Autodesk Inventor part; units mm, degrees
(part 3 of 3)
sketch "Эскиз6" plane through (0, 2, 0) normal (0, 1, 0) x (1, 0, 0)
  circle A0 centre (0, -40) radius 1.6 construction
  circle A1 centre (-46, 0) radius 1.6 construction
  circle A2 centre (46, 0) radius 1.6 construction
  line L0 (-6.2595, 46.1335) -> (-19.2746, 46.1335) construction
  arc A3 (-19.2746, 46.1335) -> (-21.6698, 47.1257) centre (-21.9203, 43.1335) ccw construction
  line L1 (-21.6698, 47.1257) -> (-42.4264, 67.8823) construction
  line L2 (-42.4264, 67.8823) -> (-34.2947, 76.014) construction
  arc A4 (-34.2947, 76.014) -> (-34.2947, 83.085) centre (-37.8302, 79.5495) ccw construction
  line L3 (-34.2947, 83.085) -> (-38.3892, 87.1795) construction
  arc A5 (-37.7453, 90.4395) -> (-38.3892, 87.1795) centre (-36.975, 88.5938) ccw construction
  arc A6 (-25.8102, 94.5401) -> (-37.7453, 90.4395) centre (0, 0) ccw construction
  arc A7 (-25.8102, 94.5401) -> (-20.7476, 95.7786) centre (-24, 98.1071) ccw construction
  arc A8 (20.7476, 95.7786) -> (-20.7476, 95.7786) centre (0, 0) ccw construction
  arc A9 (20.7476, 95.7786) -> (25.8102, 94.5401) centre (24, 98.1071) ccw construction
  arc A10 (37.7453, 90.4395) -> (25.8102, 94.5401) centre (0, 0) ccw construction
  arc A11 (38.3892, 87.1795) -> (37.7453, 90.4395) centre (36.975, 88.5938) ccw construction
  line L4 (38.3892, 87.1795) -> (34.2947, 83.085) construction
  arc A12 (34.2947, 83.085) -> (34.2947, 76.014) centre (37.8302, 79.5495) ccw construction
  line L5 (34.2947, 76.014) -> (42.4264, 67.8823) construction
  line L6 (42.4264, 67.8823) -> (21.6698, 47.1257) construction
  arc A13 (21.6698, 47.1257) -> (19.2746, 46.1335) centre (21.9203, 43.1335) ccw construction
  line L7 (19.2746, 46.1335) -> (6.2595, 46.1335) construction
  arc A14 (3.5768, 47.7906) -> (6.2595, 46.1335) centre (6.2595, 49.1335) ccw construction
  arc A15 (3.5768, 47.7906) -> (-3.5768, 47.7906) centre (0, 46) ccw construction
  arc A16 (-6.2595, 46.1335) -> (-3.5768, 47.7906) centre (-6.2595, 49.1335) ccw construction
  arc A17 (48.6481, 93.0503) -> (-48.6481, 93.0503) centre (0, 0) ccw construction
  arc A18 (-48.6481, 93.0503) -> (-49.3795, 88.2704) centre (-47.2582, 90.3917) ccw construction
  line L8 (-49.3795, 88.2704) -> (-46.3155, 85.2064) construction
  arc A19 (-46.3155, 73.8927) -> (-46.3155, 85.2064) centre (-51.9723, 79.5495) ccw construction
  line L9 (-46.3155, 73.8927) -> (-73.8927, 46.3155) construction
  arc A20 (-85.2064, 46.3155) -> (-73.8927, 46.3155) centre (-79.5495, 51.9723) ccw construction
  line L10 (-85.2064, 46.3155) -> (-88.2704, 49.3795) construction
  arc A21 (-88.2704, 49.3795) -> (-93.0503, 48.6481) centre (-90.3917, 47.2582) ccw projected
  arc A22 (-93.0503, 48.6481) -> (-93.0503, -48.6481) centre (0, 0) ccw construction
  arc A23 (-93.0503, -48.6481) -> (-88.2704, -49.3795) centre (-90.3917, -47.2582) ccw projected
  line L11 (-88.2704, -49.3795) -> (-85.2064, -46.3155) construction
  arc A24 (-73.8927, -46.3155) -> (-85.2064, -46.3155) centre (-79.5495, -51.9723) ccw construction
  line L12 (-73.8927, -46.3155) -> (-46.3155, -73.8927) construction
  arc A25 (-46.3155, -85.2064) -> (-46.3155, -73.8927) centre (-51.9723, -79.5495) ccw construction
  line L13 (-46.3155, -85.2064) -> (-49.3795, -88.2704) construction
  arc A26 (-49.3795, -88.2704) -> (-48.6481, -93.0503) centre (-47.2582, -90.3917) ccw construction
  arc A27 (-48.6481, -93.0503) -> (-45.42, -94.668) centre (0, 0) ccw construction
  arc A28 (-45.42, -94.668) -> (-43.0355, -94.1655) centre (-44.5548, -92.8648) ccw construction
  line L14 (-43.0355, -94.1655) -> (-18.3802, -65.3664) construction
  arc A29 (-17.477, -64.7643) -> (-18.3802, -65.3664) centre (-16.8609, -66.6671) ccw construction
  line L15 (-17.477, -64.7643) -> (-0.6161, -59.3045) construction
  arc A30 (0.6161, -59.3045) -> (-0.6161, -59.3045) centre (0, -61.2072) ccw construction
  line L16 (0.6161, -59.3045) -> (17.477, -64.7643) construction
  arc A31 (18.3802, -65.3664) -> (17.477, -64.7643) centre (16.8609, -66.6671) ccw construction
  line L17 (18.3802, -65.3664) -> (43.0355, -94.1655) construction
  arc A32 (43.0355, -94.1655) -> (45.42, -94.668) centre (44.5548, -92.8648) ccw construction
  arc A33 (45.42, -94.668) -> (48.6481, -93.0503) centre (0, 0) ccw construction
  arc A34 (48.6481, -93.0503) -> (49.3795, -88.2704) centre (47.2582, -90.3917) ccw construction
  line L18 (49.3795, -88.2704) -> (46.3155, -85.2064) construction
  arc A35 (46.3155, -73.8927) -> (46.3155, -85.2064) centre (51.9723, -79.5495) ccw construction
  line L19 (46.3155, -73.8927) -> (73.8927, -46.3155) construction
  arc A36 (85.2064, -46.3155) -> (73.8927, -46.3155) centre (79.5495, -51.9723) ccw construction
  line L20 (85.2064, -46.3155) -> (88.2704, -49.3795) construction
  arc A37 (88.2704, -49.3795) -> (93.0503, -48.6481) centre (90.3917, -47.2582) ccw construction
  arc A38 (93.0503, -48.6481) -> (93.0503, 48.6481) centre (0, 0) ccw construction
  arc A39 (93.0503, 48.6481) -> (88.2704, 49.3795) centre (90.3917, 47.2582) ccw construction
  line L21 (88.2704, 49.3795) -> (85.2064, 46.3155) construction
  arc A40 (73.8927, 46.3155) -> (85.2064, 46.3155) centre (79.5495, 51.9723) ccw construction
  line L22 (73.8927, 46.3155) -> (46.3155, 73.8927) construction
  arc A41 (46.3155, 85.2064) -> (46.3155, 73.8927) centre (51.9723, 79.5495) ccw construction
  line L23 (46.3155, 85.2064) -> (49.3795, 88.2704) construction
  arc A42 (49.3795, 88.2704) -> (48.6481, 93.0503) centre (47.2582, 90.3917) ccw construction
  circle A43 centre (-24, 98.1071) radius 1.6 construction
  arc A44 (47.7906, -3.5768) -> (46.1335, -6.2595) centre (49.1335, -6.2595) ccw construction
  arc A45 (47.7906, -3.5768) -> (47.7906, 3.5768) centre (46, 0) ccw construction
  arc A46 (46.1335, 6.2595) -> (47.7906, 3.5768) centre (49.1335, 6.2595) ccw construction
  line L24 (46.1335, 6.2595) -> (46.1335, 19.2746) construction
  arc A47 (46.1335, 19.2746) -> (47.1257, 21.6698) centre (43.1335, 21.9203) ccw construction
  line L25 (47.1257, 21.6698) -> (67.8823, 42.4264) construction
  line L26 (67.8823, 42.4264) -> (76.014, 34.2947) construction
  arc A48 (76.014, 34.2947) -> (83.085, 34.2947) centre (79.5495, 37.8302) ccw construction
  line L27 (83.085, 34.2947) -> (87.1795, 38.3892) construction
  arc A49 (90.4395, 37.7453) -> (87.1795, 38.3892) centre (88.5938, 36.975) ccw construction
  arc A50 (97.9653, 2.6059) -> (90.4395, 37.7453) centre (0, 0) ccw construction
  arc A51 (97.9653, 2.6059) -> (97.9653, -2.6059) centre (101, 0) ccw construction
  arc A52 (90.4395, -37.7453) -> (97.9653, -2.6059) centre (0, 0) ccw construction
  arc A53 (87.1795, -38.3892) -> (90.4395, -37.7453) centre (88.5938, -36.975) ccw construction
  line L28 (87.1795, -38.3892) -> (83.085, -34.2947) construction
  arc A54 (83.085, -34.2947) -> (76.014, -34.2947) centre (79.5495, -37.8302) ccw construction
  line L29 (76.014, -34.2947) -> (67.8823, -42.4264) construction
  line L30 (67.8823, -42.4264) -> (47.1257, -21.6698) construction
  arc A55 (47.1257, -21.6698) -> (46.1335, -19.2746) centre (43.1335, -21.9203) ccw construction
  line L31 (46.1335, -19.2746) -> (46.1335, -6.2595) construction
  circle A56 centre (101, 0) radius 1.6 construction
  circle A57 centre (-101, 0) radius 1.6 construction
  arc A58 (-47.7906, 3.5768) -> (-46.1335, 6.2595) centre (-49.1335, 6.2595) ccw construction
  arc A59 (-47.7906, 3.5768) -> (-47.7906, -3.5768) centre (-46, 0) ccw construction
  arc A60 (-46.1335, -6.2595) -> (-47.7906, -3.5768) centre (-49.1335, -6.2595) ccw construction
  line L32 (-46.1335, -6.2595) -> (-46.1335, -19.2746) construction
  arc A61 (-46.1335, -19.2746) -> (-47.1257, -21.6698) centre (-43.1335, -21.9203) ccw construction
  line L33 (-47.1257, -21.6698) -> (-67.8823, -42.4264) construction
  line L34 (-67.8823, -42.4264) -> (-76.014, -34.2947) construction
  arc A62 (-76.014, -34.2947) -> (-83.085, -34.2947) centre (-79.5495, -37.8302) ccw construction
  line L35 (-83.085, -34.2947) -> (-87.1795, -38.3892) construction
  arc A63 (-90.4395, -37.7453) -> (-87.1795, -38.3892) centre (-88.5938, -36.975) ccw construction
  arc A64 (-97.9653, -2.6059) -> (-90.4395, -37.7453) centre (0, 0) ccw construction
  arc A65 (-97.9653, -2.6059) -> (-97.9653, 2.6059) centre (-101, 0) ccw construction
  arc A66 (-90.4395, 37.7453) -> (-97.9653, 2.6059) centre (0, 0) ccw construction
  arc A67 (-87.1795, 38.3892) -> (-90.4395, 37.7453) centre (-88.5938, 36.975) ccw construction
  line L36 (-87.1795, 38.3892) -> (-83.085, 34.2947) construction
  arc A68 (-83.085, 34.2947) -> (-76.014, 34.2947) centre (-79.5495, 37.8302) ccw construction
  line L37 (-76.014, 34.2947) -> (-67.8823, 42.4264) construction
  line L38 (-67.8823, 42.4264) -> (-47.1257, 21.6698) construction
  arc A69 (-47.1257, 21.6698) -> (-46.1335, 19.2746) centre (-43.1335, 21.9203) ccw construction
  line L39 (-46.1335, 19.2746) -> (-46.1335, 6.2595) construction
  circle A70 centre (45.1111, -90.3659) radius 1.6 construction
  circle A71 centre (45.1111, 90.3659) radius 1.6 construction
  circle A72 centre (90.3659, 45.1111) radius 1.6 construction
  circle A73 centre (-45.1111, -90.3659) radius 1.6 construction
  circle A74 centre (90.3659, -45.1111) radius 1.6 construction
  circle A75 centre (-45.1111, 90.3659) radius 1.6 construction
  circle A76 centre (-90.3659, 45.1111) radius 1.6 construction
  circle A77 centre (-90.3659, -45.1111) radius 1.6 construction
  line L40 (63.6396, 46.669) -> (43.8406, 26.8701) construction
  arc A78 (41.0122, 26.8701) -> (43.8406, 26.8701) centre (42.4264, 28.2843) ccw construction
  line L41 (41.0122, 26.8701) -> (26.8701, 41.0122) construction
  arc A79 (26.8701, 43.8406) -> (26.8701, 41.0122) centre (28.2843, 42.4264) ccw construction
  line L42 (26.8701, 43.8406) -> (46.669, 63.6396) construction
  line L43 (46.669, 63.6396) -> (63.6396, 46.669) construction
  line L44 (-46.669, 63.6396) -> (-26.8701, 43.8406) construction
  arc A80 (-26.8701, 41.0122) -> (-26.8701, 43.8406) centre (-28.2843, 42.4264) ccw construction
  line L45 (-26.8701, 41.0122) -> (-41.0122, 26.8701) construction
  arc A81 (-43.8406, 26.8701) -> (-41.0122, 26.8701) centre (-42.4264, 28.2843) ccw construction
  line L46 (-43.8406, 26.8701) -> (-63.6396, 46.669) construction
  line L47 (-63.6396, 46.669) -> (-46.669, 63.6396) construction
  line L48 (-63.6396, -46.669) -> (-43.8406, -26.8701) construction
  arc A82 (-41.0122, -26.8701) -> (-43.8406, -26.8701) centre (-42.4264, -28.2843) ccw construction
  line L49 (-41.0122, -26.8701) -> (-26.8701, -41.0122) construction
  arc A83 (-26.8701, -43.8406) -> (-26.8701, -41.0122) centre (-28.2843, -42.4264) ccw construction
  line L50 (-26.8701, -43.8406) -> (-46.669, -63.6396) construction
  line L51 (-46.669, -63.6396) -> (-63.6396, -46.669) construction
  line L52 (-42.4264, -67.8823) -> (-21.6698, -47.1257) construction
  arc A84 (-21.6698, -47.1257) -> (-19.2746, -46.1335) centre (-21.9203, -43.1335) ccw construction
  line L53 (-19.2746, -46.1335) -> (19.2746, -46.1335) construction
  arc A85 (19.2746, -46.1335) -> (21.6698, -47.1257) centre (21.9203, -43.1335) ccw construction
  line L54 (21.6698, -47.1257) -> (42.4264, -67.8823) construction
  line L55 (42.4264, -67.8823) -> (37.1244, -73.1843) construction
  arc A86 (34.1909, -73.0707) -> (37.1244, -73.1843) centre (35.7102, -71.7701) ccw construction
  line L56 (34.1909, -73.0707) -> (25.4187, -62.8242) construction
  arc A87 (24.842, -61.8893) -> (25.4187, -62.8242) centre (28.1154, -60.5155) ccw construction
  line L57 (24.842, -61.8893) -> (23.8313, -59.4808) construction
  arc A88 (23.8313, -59.4808) -> (21.0049, -57.3328) centre (20.5578, -60.8546) ccw construction
  line L58 (21.0049, -57.3328) -> (15.1585, -56.5907) construction
  arc A89 (14.5119, -56.4463) -> (15.1585, -56.5907) centre (15.6055, -53.069) ccw construction
  line L59 (14.5119, -56.4463) -> (0.6161, -51.9466) construction
  arc A90 (0.6161, -51.9466) -> (-0.6161, -51.9466) centre (0, -53.8493) ccw construction
  line L60 (-0.6161, -51.9466) -> (-14.5119, -56.4463) construction
  arc A91 (-15.1585, -56.5907) -> (-14.5119, -56.4463) centre (-15.6055, -53.069) ccw construction
  line L61 (-15.1585, -56.5907) -> (-21.0049, -57.3328) construction
  arc A92 (-21.0049, -57.3328) -> (-23.8313, -59.4808) centre (-20.5578, -60.8546) ccw construction
  line L62 (-23.8313, -59.4808) -> (-24.842, -61.8893) construction
  arc A93 (-25.4187, -62.8242) -> (-24.842, -61.8893) centre (-28.1154, -60.5155) ccw construction
  line L63 (-25.4187, -62.8242) -> (-34.1909, -73.0707) construction
  arc A94 (-37.1244, -73.1843) -> (-34.1909, -73.0707) centre (-35.7102, -71.7701) ccw construction
  line L64 (-37.1244, -73.1843) -> (-42.4264, -67.8823) construction
  circle A95 centre (43.1335, 21.9203) radius 1.6 construction
  circle A96 centre (21.9203, -43.1335) radius 1.6 construction
  circle A97 centre (-21.9203, -43.1335) radius 1.6 construction
  circle A98 centre (-43.1335, -21.9203) radius 1.6 construction
  circle A99 centre (-43.1335, 21.9203) radius 1.6 construction
  circle A100 centre (-21.9203, 43.1335) radius 1.6 construction
  circle A101 centre (43.1335, -21.9203) radius 1.6 construction
  circle A102 centre (21.9203, 43.1335) radius 1.6 construction
  circle A103 centre (-37.8302, 79.5495) radius 1.6 construction
  circle A104 centre (-79.5495, 37.8302) radius 1.6 construction
  circle A105 centre (-79.5495, -37.8302) radius 1.6 construction
  circle A106 centre (79.5495, -37.8302) radius 1.6 construction
  circle A107 centre (37.8302, 79.5495) radius 1.6 construction
  circle A108 centre (79.5495, 37.8302) radius 1.6 construction
  circle A109 centre (-20.5578, -60.8546) radius 1.55 construction
  circle A110 centre (20.5578, -60.8546) radius 1.55 construction
  circle A111 centre (37.8302, -79.5495) radius 1.6 construction
  circle A112 centre (-37.8302, -79.5495) radius 1.6 construction
  line L65 (46.669, -63.6396) -> (26.8701, -43.8406) construction
  arc A113 (26.8701, -41.0122) -> (26.8701, -43.8406) centre (28.2843, -42.4264) ccw construction
  line L66 (26.8701, -41.0122) -> (41.0122, -26.8701) construction
  arc A114 (43.8406, -26.8701) -> (41.0122, -26.8701) centre (42.4264, -28.2843) ccw construction
  line L67 (43.8406, -26.8701) -> (63.6396, -46.669) construction
  line L68 (63.6396, -46.669) -> (46.669, -63.6396) construction
  circle A115 centre (24, 98.1071) radius 1.6 construction
  circle A116 centre (0, 46) radius 1.6 construction
  arc A117 (3.6492, -38.362) -> (6.3862, -40.1335) centre (6.3862, -37.1335) ccw construction
  arc A118 (3.6492, -38.362) -> (-3.6492, -38.362) centre (0, -40) ccw construction
  arc A119 (-6.3862, -40.1335) -> (-3.6492, -38.362) centre (-6.3862, -37.1335) ccw construction
  line L69 (-6.3862, -40.1335) -> (-19.2746, -40.1335) construction
  arc A120 (-19.2746, -40.1335) -> (-21.6698, -39.1414) centre (-21.9203, -43.1335) ccw construction
  line L70 (-21.6698, -39.1414) -> (-39.1414, -21.6698) construction
  arc A121 (-39.1414, -21.6698) -> (-40.1335, -19.2746) centre (-43.1335, -21.9203) ccw construction
  line L71 (-40.1335, -19.2746) -> (-40.1335, 19.2746) construction
  arc A122 (-40.1335, 19.2746) -> (-39.1414, 21.6698) centre (-43.1335, 21.9203) ccw construction
  line L72 (-39.1414, 21.6698) -> (-21.6698, 39.1414) construction
  arc A123 (-21.6698, 39.1414) -> (-19.2746, 40.1335) centre (-21.9203, 43.1335) ccw construction
  line L73 (-19.2746, 40.1335) -> (19.2746, 40.1335) construction
  arc A124 (19.2746, 40.1335) -> (21.6698, 39.1414) centre (21.9203, 43.1335) ccw construction
  line L74 (21.6698, 39.1414) -> (39.1414, 21.6698) construction
  arc A125 (39.1414, 21.6698) -> (40.1335, 19.2746) centre (43.1335, 21.9203) ccw construction
  line L75 (40.1335, 19.2746) -> (40.1335, -19.2746) construction
  arc A126 (40.1335, -19.2746) -> (39.1414, -21.6698) centre (43.1335, -21.9203) ccw construction
  line L76 (39.1414, -21.6698) -> (21.6698, -39.1414) construction
  arc A127 (21.6698, -39.1414) -> (19.2746, -40.1335) centre (21.9203, -43.1335) ccw construction
  line L77 (19.2746, -40.1335) -> (6.3862, -40.1335) construction
  arc A128 (-93.6694, -39.0933) -> (-84.7047, -40.864) centre (-88.5938, -36.975) ccw construction
  line L78 (-84.7047, -40.864) -> (-80.6102, -36.7696) construction
  arc A129 (-78.4889, -36.7696) -> (-80.6102, -36.7696) centre (-79.5495, -37.8302) ccw construction
  line L79 (-78.4889, -36.7696) -> (-67.8823, -47.3762) construction
  line L80 (-67.8823, -47.3762) -> (-42.78, -22.2739) construction
  arc A130 (-42.6335, -21.9203) -> (-42.78, -22.2739) centre (-43.1335, -21.9203) ccw construction
  line L81 (-42.6335, -21.9203) -> (-42.6335, -6.2595) construction
  line L82 (-42.6335, 6.2595) -> (-42.6335, 21.9203) construction
  arc A131 (-42.78, 22.2739) -> (-42.6335, 21.9203) centre (-43.1335, 21.9203) ccw construction
  line L83 (-42.78, 22.2739) -> (-67.8823, 47.3762) construction
  line L84 (-67.8823, 47.3762) -> (-78.4889, 36.7696) construction
  arc A132 (-80.6102, 36.7696) -> (-78.4889, 36.7696) centre (-79.5495, 37.8302) ccw construction
  line L85 (-80.6102, 36.7696) -> (-84.7047, 40.864) construction
  arc A133 (-101, -3.5) -> (-101.3693, 3.4805) centre (-101, 0) ccw
  arc A134 (-93.0503, 48.6481) -> (-93.0503, -48.6481) centre (0, 0) ccw construction
  arc A135 (-105, 0) -> (-93.0503, -48.6481) centre (0, 0) ccw
  arc A136 (-93.0503, 48.6481) -> (-105, 0) centre (0, 0) ccw
  line L86 (-88.2704, -49.3795) -> (-85.2064, -46.3155) projected
  line L87 (-90.4395, -37.7453) -> (-90.4197, -37.791)
  circle A137 centre (-101, 0) radius 1.5
  circle A138 centre (-90.3659, 45.1111) radius 1.5
  circle A139 centre (-90.3659, -45.1111) radius 1.5
  line L88 (-160.5035, 209.2939) -> (164.9125, 209.2939)
  line L89 (164.9125, 209.2939) -> (164.9125, -147.441)
  line L90 (164.9125, -147.441) -> (-160.5035, -147.441)
  line L91 (-160.5035, -147.441) -> (-160.5035, 209.2939)
  arc A140 (-89.8279, 38.5487) -> (-88.4585, -41.5951) centre (0, 0) ccw construction
  arc A141 (-93.6644, 42.8483) -> (-88.4585, 41.5951) centre (-90.3659, 45.1111) ccw
  arc A142 (-88.2704, 49.3795) -> (-93.0503, 48.6481) centre (-90.3917, 47.2582) ccw projected
  line L92 (-88.2704, 49.3795) -> (-85.7735, 46.8826)
  circle A143 centre (-46, 0) radius 1.6 construction
  line L93 (-46, 0) -> (46, 0) construction
  arc A144 (-88.4585, -41.5951) -> (-93.6644, -42.8483) centre (-90.3659, -45.1111) ccw
  arc A145 (-88.4585, 41.5951) -> (-89.8279, 38.5487) centre (0, 0) ccw construction
  arc A146 (-85.7735, 46.8826) -> (-88.4585, 41.5951) centre (0, 0) ccw
  arc A147 (-88.4585, -41.5951) -> (-85.7735, -46.8826) centre (0, 0) ccw
  arc A148 (-85.7735, -46.8826) -> (-85.7735, 46.8826) centre (0, 0) ccw construction
  arc A149 (-102.9405, -3.5) -> (-93.6644, -42.8483) centre (0, 0) ccw
  line L94 (-101, -3.5) -> (-102.9405, -3.5)
  line L95 (-46, 0) -> (-101, 0) construction
  line L96 (-101, 3.5) -> (-102.9405, 3.5)
  arc A150 (-102.9405, 3.5) -> (-102.9405, -3.5) centre (0, 0) ccw construction
  arc A151 (-93.6644, 42.8483) -> (-102.9405, 3.5) centre (0, 0) ccw
  arc A152 (-93.6644, -42.8483) -> (-93.6644, 42.8483) centre (0, 0) ccw construction
  point P0 (-101, 3.5)
  dimension "d112" = 7
  dimension "d115" = 105
  dimension "d116" = 105
  dimension "d119" = 3
  dimension "d120" = 3
  dimension "d121" = 3
  dimension "d126" = 195.5
  dimension "d128" = 4
  dimension "d139" = 2
  constraints: 44 point on circle, 36 end point, 22 centre point, 6 coincident, 4 symmetric about line, 3 horizontal, 3 parallel, 2 point on line, 1 perpendicular, 1 tangent, 12 other
  measures "d112" diameter of A133
  measures "d115" radius of A135
  measures "d116" radius of A136
  measures "d119" diameter of A137
  measures "d120" diameter of A138
  measures "d121" diameter of A139
  measures "d126" diameter of A140
  measures "d128" radius of A141
  measures "d139" radial gap between concentric circles of A22 A149
extrude "Выдавливание9" add sketch "Эскиз6" along normal blind 35 contours L92 A146 A141 A151 L96 A133 L94 A149 A144 A147 L86 A23 A135 A136 A21
extrude "Выдавливание10" cut sketch "Эскиз6" against normal blind 10 contours L92 A146 A141 A151 L96 A133 L94 A149 A144 A147 L86 A23 A135 A136 A21 | A137 | A138 | A139 | L88 L89 L90 L91
fillet "Сопряжение1" radius 2 4 edges at (-85.7735, 19.5, -46.8826) (-85.7735, 19.5, 46.8826) (-88.4585, 19.5, 41.5951) (-88.4585, 19.5, -41.5951)
ref_plane "РабПлоскость2" through (-105, 2, 0) normal (1, 0, 0) x (0, 1, 0)
ref_plane "РабПлоскость3" through (-86.4693, 2, -45.5865) normal (-1, 0, 0) x (0, -1, 0)
sketch "Эскиз10" plane through (0, 0, 0) normal (0, 0, 1) x (1, 0, 0)
  line L0 (-97.5, 2) -> (-97.5, 37) construction
  line L1 (-109.4804, 30.0716) -> (-60.859, 2) construction
  line L2 (-89.4935, 2) -> (-88.1266, 2) construction
  line L3 (-89.4935, 2) -> (-93.6644, 2) construction
  line L4 (-93.6644, 2) -> (-102.9405, 2) construction
  line L5 (-102.9405, 2) -> (-101, 2) construction
  line L6 (-101, 2) -> (-101, 2) construction
  line L7 (-101, 2) -> (-102.9405, 2) construction
  line L8 (-102.9405, 2) -> (-93.6644, 2) construction
  line L9 (-93.6644, 2) -> (-89.4935, 2) construction
  line L10 (-88.1266, 2) -> (-89.4935, 2) construction
  line L11 (-88.1266, 2) -> (-86.4693, 2) construction
  line L12 (-86.8243, 2) -> (-86.4693, 2) construction
  line L13 (-88.2704, 2) -> (-86.8243, 2) construction
  line L14 (-93.0503, 2) -> (-88.2704, 2) construction
  line L15 (-93.0503, 2) -> (-93.0503, 2) construction
  line L16 (-88.2704, 2) -> (-93.0503, 2) construction
  line L17 (-86.8243, 2) -> (-88.2704, 2) construction
  line L18 (-86.4693, 2) -> (-86.8243, 2) construction
  line L19 (-86.4693, 2) -> (-88.1266, 2) construction
  line L20 (-102.5, 2) -> (-99.5, 2) construction
  line L21 (-91.8659, 2) -> (-88.8659, 2) construction
  line L22 (-91.8659, 2) -> (-88.8659, 2) construction
  line L23 (-64.3231, 4) -> (-95.5, 22)
  point P0 (0, 0)
  dimension "d157" = 60
  dimension "d158" = 11.9904
  dimension "d197" = 2
  dimension "d198" = 36
  dimension "d199" = 2
  constraints: 4 end point, 3 point on line
  measures "d157" angle of L0 L1
  measures "d158" distance from line of L0.end L1
  measures "d197" distance from line of L4 L23.start
  measures "d198" distance of L23.start L23.end
  measures "d199" distance from line of L0 L23.end
sketch "Эскиз11" plane through (-86.4693, 2, -45.5865) normal (-1, 0, 0) x (0, -1, 0)
  line L0 (-33.2, 80.5865) -> (-2, 80.5865)
  line L1 (-2, 80.5865) -> (-2, 10.5865)
  line L2 (-2, 10.5865) -> (-33.2, 10.5865)
  line L3 (-33.2, 10.5865) -> (-33.2, 80.5865)
  line L4 (-33.2, 45.5865) -> (-2, 45.5865) construction
  line L5 (-17.6, 10.5865) -> (-17.6, 80.5865) construction
  line L6 (-35, 44.0865) -> (-35, 47.0865) construction
  line L7 (0, 44.0865) -> (0, 47.0865) construction
  line L8 (0, 45.5865) -> (-35, 45.5865) construction
  point P0 (2, 45.5865)
  dimension "d154" = 70
  dimension "d155" = 31.2
  dimension "d156" = 2
  constraints: 14 end point, 6 midpoint, 2 parallel, 1 collinear, 1 horizontal, 1 perpendicular
  measures "d154" distance of L2.end L0.start
  measures "d155" distance of L1.end L2.end
  measures "d156" distance between parallel lines of L7 L1
ref_plane "РабПлоскость4" through (-109.4804, 30.0716, 0) normal (0.5, 0.8660254, 0) x (0.8660254, -0.5, 0)
ref_plane "РабПлоскость5" through (0, 2, 0) normal (0, -1, 0) x (1, 0, 0)
ref_plane "РабПлоскость6" through (0, 37, 0) normal (0, 1, 0) x (1, 0, 0)
sketch "Эскиз12" plane through (-109.4804, 30.0716, 0) normal (0.5, 0.8660254, 0) x (0.8660254, -0.5, 0)
  line L0 (16.1432, -35) -> (52.1432, -35) construction
  line L1 (52.1432, -35) -> (52.1432, 35.3) construction
  line L2 (52.1432, 35.3) -> (16.1432, 35.3) construction
  line L3 (16.1432, 35.3) -> (16.1432, -35) construction
  ellipse E0 centre (3.88, 0) end of major axis (3.88, 1.5) minor radius 1.299 construction
  ellipse E1 centre (13.0894, -45.1111) end of major axis (13.0894, -43.6111) minor radius 1.299 construction
  ellipse E2 centre (13.0894, 45.1111) end of major axis (13.0894, 46.6111) minor radius 1.299 construction
  ellipse E3 centre (13.4672, 43.1592) end of major axis (13.4672, 41.1592) minor radius 1.7321 (13.845, 41.2074) -> (15.0287, 42.2939) ccw construction
  ellipse E4 centre (91.3486, 0) end of major axis (91.3486, -97.75) minor radius 84.654 (16.464, 45.5865) -> (15.0287, 42.2939) ccw construction
  ellipse E5 centre (14.9318, 46.5192) end of major axis (14.9318, 44.5192) minor radius 1.7321 (16.464, 45.5865) -> (16.1566, 47.9334) ccw construction
  line L4 (16.1566, 47.9334) -> (14.9042, 49.3795) construction
  ellipse E6 centre (13.0671, 47.2582) end of major axis (13.0671, 50.2582) minor radius 2.5981 (14.9042, 49.3795) -> (10.7647, 48.6481) ccw construction
  ellipse E7 centre (91.3486, 0) end of major axis (91.3486, -105) minor radius 90.9327 (10.7647, 48.6481) -> (10.7647, -48.6481) ccw construction
  ellipse E8 centre (13.0671, -47.2582) end of major axis (13.0671, -50.2582) minor radius 2.5981 (10.7647, -48.6481) -> (14.9042, -49.3795) ccw construction
  line L5 (14.9042, -49.3795) -> (16.1566, -47.9334) construction
  ellipse E9 centre (14.9318, -46.5192) end of major axis (14.9318, -48.5192) minor radius 1.7321 (16.1566, -47.9334) -> (16.464, -45.5865) ccw construction
  ellipse E10 centre (91.3486, 0) end of major axis (91.3486, -97.75) minor radius 84.654 (15.0287, -42.2939) -> (16.464, -45.5865) ccw construction
  ellipse E11 centre (13.4672, -43.1592) end of major axis (13.4672, -45.1592) minor radius 1.7321 (15.0287, -42.2939) -> (13.845, -41.2074) ccw construction
  ellipse E12 centre (13.0894, -45.1111) end of major axis (13.0894, -41.1111) minor radius 3.4641 (13.845, -41.2074) -> (10.2328, -42.8483) ccw construction
  ellipse E13 centre (91.3486, 0) end of major axis (91.3486, -103) minor radius 89.2006 (2.1995, -3.5) -> (10.2328, -42.8483) ccw construction
  line L6 (2.1995, -3.5) -> (3.88, -3.5) construction
  ellipse E14 centre (3.88, 0) end of major axis (3.88, -3.5) minor radius 3.0311 (3.88, -3.5) -> (3.88, 3.5) ccw construction
  line L7 (3.88, 3.5) -> (2.1995, 3.5) construction
  ellipse E15 centre (91.3486, 0) end of major axis (91.3486, -103) minor radius 89.2006 (10.2328, 42.8483) -> (2.1995, 3.5) ccw construction
  ellipse E16 centre (13.0894, 45.1111) end of major axis (13.0894, 41.1111) minor radius 3.4641 (10.2328, 42.8483) -> (13.845, 41.2074) ccw construction
  ellipse E17 centre (91.3486, 0) end of major axis (91.3486, -105) minor radius 90.9327 (10.7647, 48.6481) -> (10.7647, -48.6481) ccw construction
  ellipse E18 centre (91.3486, 0) end of major axis (91.3486, -103) minor radius 89.2006 (2.1995, -3.5) -> (10.2328, -42.8483) ccw construction
  ellipse E19 centre (91.3486, 0) end of major axis (91.3486, -103) minor radius 89.2006 (10.2328, 42.8483) -> (2.1995, 3.5) ccw construction
  line L8 (-13.8568, 77.6335) -> (-13.8568, -83.7272) construction
  line L9 (56.1432, 77.6335) -> (56.1432, -83.7272) construction
  line L10 (16.1432, 0.15) -> (52.1432, 0.15) construction
  line L11 (0, 0) -> (56.1432, 0) construction
  circle A0 centre (18.6432, -31) radius 1.9
  line L12 (34.1432, -35) -> (34.1432, 35.3) construction
  circle A1 centre (49.6432, -31) radius 1.9
  circle A2 centre (18.7682, 31.05) radius 1.9
  circle A3 centre (49.5182, 31.05) radius 1.9
  line L13 (16.6432, -35) -> (20.6432, -35)
  line L14 (22.6432, -33) -> (22.6432, -29)
  line L15 (20.6432, -27) -> (16.6432, -27)
  line L16 (14.6432, -29) -> (14.6432, -33)
  arc A4 (20.6432, -35) -> (22.6432, -33) centre (20.6432, -33) ccw
  arc A5 (14.6432, -33) -> (16.6432, -35) centre (16.6432, -33) ccw
  arc A6 (16.6432, -27) -> (14.6432, -29) centre (16.6432, -29) ccw
  arc A7 (22.6432, -29) -> (20.6432, -27) centre (20.6432, -29) ccw
  line L17 (51.6432, -35) -> (47.6432, -35)
  line L18 (45.6432, -33) -> (45.6432, -29)
  line L19 (47.6432, -27) -> (51.6432, -27)
  arc A8 (45.6432, -33) -> (47.6432, -35) centre (47.6432, -33) ccw
  arc A9 (51.6432, -35) -> (53.6432, -33) centre (51.6432, -33) ccw
  arc A10 (53.6432, -29) -> (51.6432, -27) centre (51.6432, -29) ccw
  arc A11 (47.6432, -27) -> (45.6432, -29) centre (47.6432, -29) ccw
  line L20 (53.6432, -29) -> (53.6432, -33)
  line L21 (16.7682, 27.05) -> (20.7682, 27.05)
  line L22 (22.7682, 29.05) -> (22.7682, 33.05)
  line L23 (20.7682, 35.05) -> (16.7682, 35.05)
  line L24 (14.7682, 33.05) -> (14.7682, 29.05)
  arc A12 (20.7682, 27.05) -> (22.7682, 29.05) centre (20.7682, 29.05) ccw
  arc A13 (22.7682, 33.05) -> (20.7682, 35.05) centre (20.7682, 33.05) ccw
  arc A14 (16.7682, 35.05) -> (14.7682, 33.05) centre (16.7682, 33.05) ccw
  arc A15 (14.7682, 29.05) -> (16.7682, 27.05) centre (16.7682, 29.05) ccw
  line L25 (51.5182, 27.05) -> (47.5182, 27.05)
  line L26 (45.5182, 29.05) -> (45.5182, 33.05)
  line L27 (47.5182, 35.05) -> (51.5182, 35.05)
  line L28 (53.5182, 33.05) -> (53.5182, 29.05)
  arc A16 (45.5182, 29.05) -> (47.5182, 27.05) centre (47.5182, 29.05) ccw
  arc A17 (47.5182, 35.05) -> (45.5182, 33.05) centre (47.5182, 33.05) ccw
  arc A18 (53.5182, 33.05) -> (51.5182, 35.05) centre (51.5182, 33.05) ccw
  arc A19 (51.5182, 27.05) -> (53.5182, 29.05) centre (51.5182, 29.05) ccw
  point P0 (109.8486, 0)
  point P1 (17.1354, -60.6757)
  point P2 (15.6921, -54.5631)
  point P3 (15.7023, 54.582)
  point P4 (18.6432, -32.9)
  point P5 (18.7682, 32.95)
  point P6 (22.7682, 35.05)
  point P7 (22.7682, 27.05)
  point P8 (14.7682, 35.05)
  dimension "d166" = 3.8
  dimension "d169" = 3.8
  dimension "d160" = 36
  dimension "d161" = 70.3
  dimension "d164" = 4
  dimension "d165" = 0.15
  dimension "d167" = 31
  dimension "d168" = 4
  dimension "d170" = 30.75
  dimension "d171" = 4.25
  dimension "d172" = 4
  dimension "d173" = 4
  dimension "d174" = 4
  dimension "d175" = 4
  dimension "d176" = 2
  dimension "d177" = 8
  dimension "d178" = 8
  dimension "d179" = 4
  dimension "d180" = 4
  dimension "d181" = 2
  dimension "d182" = 2
  constraints: 44 end point, 32 point on circle, 26 symmetric about line, 18 centre point, 16 tangent, 6 parallel, 6 point on line, 5 equal radius, 4 midpoint, 3 horizontal, 3 perpendicular, 2 vertical alignment, 36 other
  measures "d160" distance of L1.end L2.end
  measures "d161" distance of L2.end L0.start
  measures "d164" distance between parallel lines of L9 L1
  measures "d165" distance between parallel lines of L11 L10
  measures "d167" distance of A1.centre point (18.643, -31)
  measures "d168" distance from line of L0 point (18.643, -31)
  measures "d170" distance of A3.centre point (18.768, 31.05)
  measures "d171" distance from line of L2 point (18.768, 31.05)
  measures "d172" distance from line of point (18.643, -31) L15
  measures "d173" distance from line of point (18.643, -31) L13
  measures "d174" distance from line of point (18.643, -31) L16
  measures "d175" distance from line of point (18.643, -31) L14
  measures "d176" radius of A4
  measures "d177" distance of point (14.768, 35.05) point (22.768, 35.05)
  measures "d178" distance of point (22.768, 35.05) point (22.768, 27.05)
  measures "d179" distance from line of L24 point (18.768, 31.05)
  measures "d180" distance from line of L21 point (18.768, 31.05)
  measures "d181" radius of A12
  measures "d182" radius of A15
extrude "Выдавливание12" add sketch "Эскиз12" against normal blind 4
sketch "Эскиз8" plane through (-105, 2, 0) normal (1, 0, 0) x (0, 1, 0)
  line L0 (0, -48.6481) -> (0, 48.6481) construction
  line L1 (0, 48.6481) -> (35, 48.6481) construction
  line L2 (35, -48.6481) -> (35, 48.6481) construction
  line L3 (0, -48.6481) -> (35, -48.6481) construction
  line L4 (0, 48.6481) -> (0, 49.3795) construction
  line L5 (0, 49.3795) -> (35, 49.3795) construction
  line L6 (35, 48.6481) -> (35, 49.3795) construction
  line L7 (0, 48.6481) -> (35, 48.6481) construction
  line L8 (0, -49.3795) -> (0, -48.6481) construction
  line L9 (0, -48.6481) -> (35, -48.6481) construction
  line L10 (35, -49.3795) -> (35, -48.6481) construction
  line L11 (0, -49.3795) -> (35, -49.3795) construction
  line L12 (0, -48.6481) -> (35, -48.6481) construction
  line L13 (0, 48.6481) -> (35, 48.6481) construction
  line L14 (35, -48.6481) -> (0, 48.6481) construction
  line L15 (35, 48.6481) -> (0, -48.6481) construction
  line L16 (11.701, 7.0442) -> (20.701, -8.5442)
  line L17 (20.701, -8.5442) -> (23.299, -7.0442)
  line L18 (23.299, -7.0442) -> (14.299, 8.5442)
  line L19 (14.299, 8.5442) -> (11.701, 7.0442)
  line L20 (11.701, 7.0442) -> (23.299, -7.0442) construction
  line L21 (20.701, -8.5442) -> (14.299, 8.5442) construction
  line L22 (35, -48.6481) -> (35, 48.6481) construction
  line L23 (35, 0) -> (0, 0) construction
  line L24 (11.701, -7.0442) -> (14.299, -8.5442)
  line L25 (23.299, 7.0442) -> (20.701, 8.5442)
  line L26 (20.701, 8.5442) -> (11.701, -7.0442)
  line L27 (14.299, -8.5442) -> (20.701, 8.5442) construction
  line L28 (23.299, 7.0442) -> (11.701, -7.0442) construction
  line L29 (14.299, -8.5442) -> (23.299, 7.0442)
  line L30 (26.5, -1.5) -> (26.5, 1.5)
  line L31 (8.5, 1.5) -> (8.5, -1.5)
  line L32 (8.5, -1.5) -> (26.5, -1.5)
  line L33 (26.5, 1.5) -> (8.5, -1.5) construction
  line L34 (8.5, 1.5) -> (26.5, -1.5) construction
  line L35 (26.5, 1.5) -> (8.5, 1.5)
  point P0 (-2, 0)
  point P1 (17.5, 0)
  point P2 (17.5, 0)
  point P3 (17.5, 0)
  point P4 (14.9019, 1.5)
  point P5 (14.9019, -1.5)
  point P6 (17.5, -3)
  point P7 (20.0981, -1.5)
  point P8 (20.0981, 1.5)
  point P9 (17.5, 3)
  dimension "d143" = 3
  dimension "d144" = 18
  dimension "d145" = 60
  dimension "d148" = 360
  constraints: 42 end point, 9 midpoint, 2 coincident, 2 parallel, 1 perpendicular, 32 other
  measures "d143" distance of L17.end L16.end
  measures "d144" distance of L17.end L18.end
  measures "d145" angle of L23 L18
extrude "asterisk" cut sketch "Эскиз8" along normal blind 0.6
ref_plane "РабПлоскость7" through (-96.799, 22.75, 31) normal (1, 0, 0) x (0, 1, 0)
sketch "Эскиз13" plane through (-96.799, 22.75, 31) normal (1, 0, 0) x (0, 1, 0)
  ellipse E0 centre (-1, -2) end of major axis (-1, -4) minor radius 1 (-1, -4) -> (0, -2) ccw projected
  line L0 (0, -2) -> (0, 2) projected
  ellipse E1 centre (-1, 2) end of major axis (-1, 4) minor radius 1 (0, 2) -> (-1, 4) ccw projected
  line L1 (-1, 4) -> (-3, 4) projected
  ellipse E2 centre (-3, 2) end of major axis (-3, 4) minor radius 1 (-3, 4) -> (-4, 2) ccw construction
  line L2 (-4, 2) -> (-4, -2) construction
  ellipse E3 centre (-3, -2) end of major axis (-3, -4) minor radius 1 (-4, -2) -> (-3, -4) ccw construction
  line L3 (-3, -4) -> (-1, -4) projected
  ellipse E4 centre (-2, 0) end of major axis (-2, -1.9) minor radius 0.95 construction
  ellipse E5 centre (-16.5, -2) end of major axis (-16.5, -4) minor radius 1 (-16.5, -4) -> (-15.5, -2) ccw projected
  line L4 (-15.5, -2) -> (-15.5, 2) projected
  ellipse E6 centre (-16.5, 2) end of major axis (-16.5, 4) minor radius 1 (-15.5, 2) -> (-16.5, 4) ccw projected
  line L5 (-16.5, 4) -> (-18.5, 4) projected
  ellipse E7 centre (-18.5, 2) end of major axis (-18.5, 4) minor radius 1 (-18.5, 4) -> (-19.5, 2) ccw projected
  line L6 (-19.5, 2) -> (-19.5, -2) projected
  ellipse E8 centre (-18.5, -2) end of major axis (-18.5, -4) minor radius 1 (-19.5, -2) -> (-18.5, -4) ccw projected
  line L7 (-18.5, -4) -> (-16.5, -4) projected
  ellipse E9 centre (-17.5, 0) end of major axis (-17.5, -1.9) minor radius 0.95 construction
  line L8 (-19.5, 2) -> (-19.5, -2) construction
  line L9 (-19.5, 2) -> (-22.9641, 2) construction
  line L10 (-22.9641, -2) -> (-22.9641, 2) projected
  line L11 (-19.5, -2) -> (-22.9641, -2) construction
  ellipse E10 centre (-18.5, -2) end of major axis (-18.5, -4) minor radius 1 (-19.5, -2) -> (-18.5, -4) ccw construction
  line L12 (-19.5, -2) -> (-22.9641, -2) construction
  ellipse E11 centre (-21.9641, -2) end of major axis (-21.9641, 0) minor radius 1 (-22.9641, -2) -> (-21.9641, -4) ccw projected
  line L13 (-18.5, -4) -> (-21.9641, -4) projected
  ellipse E12 centre (-18.5, 2) end of major axis (-18.5, 4) minor radius 1 (-18.5, 4) -> (-19.5, 2) ccw construction
  line L14 (-18.5, 4) -> (-21.9641, 4) projected
  ellipse E13 centre (-21.9641, 2) end of major axis (-21.9641, 4) minor radius 1 (-21.9641, 4) -> (-22.9641, 2) ccw projected
  line L15 (-19.5, 2) -> (-22.9641, 2) construction
  ellipse E14 centre (-3, 2) end of major axis (-3, 4) minor radius 1 (-3, 4) -> (-4, 2) ccw construction
  line L16 (-3, 4) -> (-6.4641, 4) projected
  ellipse E15 centre (-6.4641, 2) end of major axis (-6.4641, 4) minor radius 1 (-6.4641, 4) -> (-7.4641, 2) ccw projected
  line L17 (-4, 2) -> (-7.4641, 2) construction
  line L18 (-4, 2) -> (-4, -2) construction
  line L19 (-4, 2) -> (-7.4641, 2) construction
  line L20 (-7.4641, -2) -> (-7.4641, 2) projected
  line L21 (-4, -2) -> (-7.4641, -2) construction
  ellipse E16 centre (-3, -2) end of major axis (-3, -4) minor radius 1 (-4, -2) -> (-3, -4) ccw construction
  line L22 (-4, -2) -> (-7.4641, -2) construction
  ellipse E17 centre (-6.4641, -2) end of major axis (-6.4641, 0) minor radius 1 (-7.4641, -2) -> (-6.4641, -4) ccw projected
  line L23 (-3, -4) -> (-6.4641, -4) projected
  ellipse E18 centre (-3.0625, -64.05) end of major axis (-3.0625, -66.05) minor radius 1 (-4.0625, -64.05) -> (-3.0625, -66.05) ccw construction
  line L24 (-3.0625, -66.05) -> (-1.0625, -66.05) projected
  ellipse E19 centre (-1.0625, -64.05) end of major axis (-1.0625, -66.05) minor radius 1 (-1.0625, -66.05) -> (-0.0625, -64.05) ccw projected
  line L25 (-0.0625, -64.05) -> (-0.0625, -60.05) projected
  ellipse E20 centre (-1.0625, -60.05) end of major axis (-1.0625, -58.05) minor radius 1 (-0.0625, -60.05) -> (-1.0625, -58.05) ccw projected
  line L26 (-1.0625, -58.05) -> (-3.0625, -58.05) projected
  ellipse E21 centre (-3.0625, -60.05) end of major axis (-3.0625, -58.05) minor radius 1 (-3.0625, -58.05) -> (-4.0625, -60.05) ccw construction
  line L27 (-4.0625, -60.05) -> (-4.0625, -64.05) construction
  ellipse E22 centre (-2.0625, -62.05) end of major axis (-2.0625, -63.95) minor radius 0.95 construction
  line L28 (-4.0625, -60.05) -> (-4.0625, -64.05) construction
  line L29 (-4.0625, -60.05) -> (-7.5266, -60.05) construction
  line L30 (-7.5266, -64.05) -> (-7.5266, -60.05) projected
  line L31 (-4.0625, -64.05) -> (-7.5266, -64.05) construction
  ellipse E23 centre (-3.0625, -60.05) end of major axis (-3.0625, -58.05) minor radius 1 (-3.0625, -58.05) -> (-4.0625, -60.05) ccw construction
  line L32 (-3.0625, -58.05) -> (-6.5266, -58.05) projected
  ellipse E24 centre (-6.5266, -60.05) end of major axis (-6.5266, -58.05) minor radius 1 (-6.5266, -58.05) -> (-7.5266, -60.05) ccw projected
  line L33 (-4.0625, -60.05) -> (-7.5266, -60.05) construction
  ellipse E25 centre (-3.0625, -64.05) end of major axis (-3.0625, -66.05) minor radius 1 (-4.0625, -64.05) -> (-3.0625, -66.05) ccw construction
  line L34 (-4.0625, -64.05) -> (-7.5266, -64.05) construction
  ellipse E26 centre (-6.5266, -64.05) end of major axis (-6.5266, -62.05) minor radius 1 (-7.5266, -64.05) -> (-6.5266, -66.05) ccw projected
  line L35 (-3.0625, -66.05) -> (-6.5266, -66.05) projected
  ellipse E27 centre (-16.4375, -60.05) end of major axis (-16.4375, -58.05) minor radius 1 (-15.4375, -60.05) -> (-16.4375, -58.05) ccw projected
  line L36 (-16.4375, -58.05) -> (-18.4375, -58.05) projected
  ellipse E28 centre (-18.4375, -60.05) end of major axis (-18.4375, -58.05) minor radius 1 (-18.4375, -58.05) -> (-19.4375, -60.05) ccw projected
  line L37 (-19.4375, -60.05) -> (-19.4375, -64.05) projected
  ellipse E29 centre (-18.4375, -64.05) end of major axis (-18.4375, -66.05) minor radius 1 (-19.4375, -64.05) -> (-18.4375, -66.05) ccw projected
  line L38 (-18.4375, -66.05) -> (-16.4375, -66.05) projected
  ellipse E30 centre (-16.4375, -64.05) end of major axis (-16.4375, -66.05) minor radius 1 (-16.4375, -66.05) -> (-15.4375, -64.05) ccw projected
  line L39 (-15.4375, -64.05) -> (-15.4375, -60.05) projected
  ellipse E31 centre (-17.4375, -62.05) end of major axis (-17.4375, -63.95) minor radius 0.95 construction
  ellipse E32 centre (-18.4375, -64.05) end of major axis (-18.4375, -66.05) minor radius 1 (-19.4375, -64.05) -> (-18.4375, -66.05) ccw construction
  line L40 (-19.4375, -64.05) -> (-22.9016, -64.05) construction
  ellipse E33 centre (-21.9016, -64.05) end of major axis (-21.9016, -62.05) minor radius 1 (-22.9016, -64.05) -> (-21.9016, -66.05) ccw projected
  line L41 (-18.4375, -66.05) -> (-21.9016, -66.05) projected
  line L42 (-19.4375, -60.05) -> (-19.4375, -64.05) construction
  line L43 (-19.4375, -60.05) -> (-19.4375, -64.05) construction
  line L44 (-19.4375, -60.05) -> (-22.9016, -60.05) construction
  line L45 (-22.9016, -64.05) -> (-22.9016, -60.05) construction
  line L46 (-19.4375, -64.05) -> (-22.9016, -64.05) construction
  ellipse E34 centre (-18.4375, -60.05) end of major axis (-18.4375, -58.05) minor radius 1 (-18.4375, -58.05) -> (-19.4375, -60.05) ccw construction
  line L47 (-18.4375, -58.05) -> (-21.9016, -58.05) projected
  ellipse E35 centre (-21.9016, -60.05) end of major axis (-21.9016, -58.05) minor radius 1 (-21.9016, -58.05) -> (-22.9016, -60.05) ccw projected
  line L48 (-19.4375, -60.05) -> (-22.9016, -60.05) construction
  ellipse E36 centre (-19.9641, -2) end of major axis (-19.9641, -4) minor radius 1 (-19.9641, -4) -> (-18.9641, -2) ccw construction
  line L49 (-19.9641, -4) -> (-21.9641, -4) construction
  ellipse E37 centre (-21.9641, -2) end of major axis (-21.9641, 0) minor radius 1 (-22.9641, -2) -> (-21.9641, -4) ccw construction
  line L50 (-22.9641, -2) -> (-22.9641, 2) construction
  ellipse E38 centre (-21.9641, 2) end of major axis (-21.9641, 4) minor radius 1 (-21.9641, 4) -> (-22.9641, 2) ccw construction
  line L51 (-21.9641, 4) -> (-19.9641, 4) construction
  ellipse E39 centre (-19.9641, 2) end of major axis (-19.9641, 0) minor radius 1 (-18.9641, 2) -> (-19.9641, 4) ccw construction
  line L52 (-18.9641, 2) -> (-18.9641, -2) construction
  ellipse E40 centre (-20.9641, 0) end of major axis (-20.9641, 1.9) minor radius 0.95 construction
  ellipse E41 centre (-19.9016, -60.05) end of major axis (-19.9016, -62.05) minor radius 1 (-18.9016, -60.05) -> (-19.9016, -58.05) ccw construction
  line L53 (-18.9016, -60.05) -> (-18.9016, -64.05) construction
  ellipse E42 centre (-19.9016, -64.05) end of major axis (-19.9016, -66.05) minor radius 1 (-19.9016, -66.05) -> (-18.9016, -64.05) ccw construction
  line L54 (-19.9016, -66.05) -> (-21.9016, -66.05) construction
  ellipse E43 centre (-21.9016, -64.05) end of major axis (-21.9016, -62.05) minor radius 1 (-22.9016, -64.05) -> (-21.9016, -66.05) ccw construction
  line L55 (-22.9016, -64.05) -> (-22.9016, -60.05) projected
  ellipse E44 centre (-21.9016, -60.05) end of major axis (-21.9016, -58.05) minor radius 1 (-21.9016, -58.05) -> (-22.9016, -60.05) ccw construction
  line L56 (-21.9016, -58.05) -> (-19.9016, -58.05) construction
  ellipse E45 centre (-20.9016, -62.05) end of major axis (-20.9016, -60.15) minor radius 0.95 construction
  ellipse E46 centre (-5.4641, 0) end of major axis (-5.4641, 1.9) minor radius 0.95 construction
  line L57 (-3.4641, -1.8839) -> (-3.4641, -2) construction
  ellipse E47 centre (-4.4641, -2) end of major axis (-4.4641, -4) minor radius 1 (-4.4641, -4) -> (-3.4641, -2) ccw construction
  line L58 (-4.4641, -4) -> (-6.4641, -4) construction
  ellipse E48 centre (-6.4641, -2) end of major axis (-6.4641, 0) minor radius 1 (-7.4641, -2) -> (-6.4641, -4) ccw construction
  line L59 (-7.4641, -2) -> (-7.4641, 2) construction
  ellipse E49 centre (-6.4641, 2) end of major axis (-6.4641, 4) minor radius 1 (-6.4641, 4) -> (-7.4641, 2) ccw construction
  line L60 (-6.4641, 4) -> (-4.5772, 4) projected
  ellipse E50 centre (-5.5266, -62.05) end of major axis (-5.5266, -60.15) minor radius 0.95 construction
  line L61 (-4.5877, -66.05) -> (-6.5266, -66.05) projected
  ellipse E51 centre (-6.5266, -64.05) end of major axis (-6.5266, -62.05) minor radius 1 (-7.5266, -64.05) -> (-6.5266, -66.05) ccw construction
  line L62 (-7.5266, -64.05) -> (-7.5266, -60.05) construction
  ellipse E52 centre (-6.5266, -60.05) end of major axis (-6.5266, -58.05) minor radius 1 (-6.5266, -58.05) -> (-7.5266, -60.05) ccw construction
  line L63 (-6.5266, -58.05) -> (-4.5266, -58.05) projected
  ellipse E53 centre (-4.5266, -60.05) end of major axis (-4.5266, -62.05) minor radius 1 (-3.5266, -60.05) -> (-4.5266, -58.05) ccw construction
  line L64 (-3.5266, -60.05) -> (-3.5266, -60.481) construction
  line L65 (-20.75, -27.5) -> (-20.75, 11.8483) projected
  line L66 (-20.75, -73.8483) -> (-20.75, -34.5) projected
  ellipse E54 centre (-60.5058, -31) end of major axis (-60.5058, -134) minor radius 59.4671 (-4.5877, -66.05) -> (-3.5266, -60.481) ccw construction
  ellipse E55 centre (-60.5058, -31) end of major axis (-60.5058, -134) minor radius 59.4671 (-3.4641, -1.8839) -> (-4.5772, 4) ccw construction
  point P0 (-22.75, -31)
  point P1 (-30.4706, -58.05)
  point P2 (-30.4706, -66.05)
  point P3 (-30.5788, -4)
  point P4 (-30.5788, 4)
  point P5 (-22.9641, 2)
  point P6 (-22.9641, -2)
  point P7 (-34.208, -3.9909)
  point P8 (-34.208, 3.9909)
  point P9 (-22.9016, -60.05)
  point P10 (-22.9016, -64.05)
  point P11 (-34.208, -66.0249)
  point P12 (-34.208, -58.0751)
  point P13 (-7.5266, -64.05)
  point P14 (-6.5266, -66.05)
  point P15 (-5.3044, -66.05)
  point P16 (-5.3044, -58.05)
  point P17 (-6.5266, -58.05)
  point P18 (-7.5266, -60.05)
  point P19 (-5.1962, 4)
  point P20 (-6.4641, 4)
  point P21 (-7.4641, 2)
  point P22 (-7.4641, -2)
  point P23 (-20.75, -4)
  point P24 (-20.75, 4)
  point P25 (-20.75, -66.05)
  point P26 (-20.75, -58.05)
  constraints: 52 other
extrude "Выдавливание13" add sketch "Эскиз13" along normal blind 28 and the other way blind 8 contours L7 E8 L6 E7 L5 E6 L4 E5 | L13 L65 L14 E7 L6 E8 | L39 E30 L38 E29 L37 E28 L36 E27 | E28 L37 E29 L41 L66 L47
extrude "Выдавливание14" cut sketch "Эскиз13" along normal blind 20 contours L13 E11 L10 E13 L14 L65 | L66 L41 E33 L55 E35 L47
extrude "Выдавливание15" add sketch "Эскиз13" along normal blind 4.92 and the other way blind 10 contours L3 L23 E17 L20 E15 L16 L1 E1 L0 E0 | L35 E26 L30 E24 L32 L26 E20 L25 E19 L24
sketch "Эскиз14" plane through (0, 37, 0) normal (0, 1, 0) x (1, 0, 0)
  arc A0 (-93.0503, 48.6481) -> (-93.0503, -48.6481) centre (0, 0) ccw projected
  arc A1 (-93.0503, 48.6481) -> (-93.0503, -48.6481) centre (0, 0) ccw projected
  line L0 (-96.9579, 40.3009) -> (-125.5201, 38.6092)
  line L1 (-125.5201, 38.6092) -> (-122.2809, -45.4761)
  line L2 (-122.2809, -45.4761) -> (-97.2, -39.7136)
  constraints: 6 end point, 2 point on circle
extrude "Выдавливание17" cut sketch "Эскиз14" against normal blind 36
extrude "Выдавливание18" cut sketch "Эскиз12" along normal blind 4.92 contours A0 | A1 | A2 | A5 L16 A6 L15 A7 L14 A4 L13 | L17 A8 L18 A11 L19 A10 L20 A9 | A15 L24 A14 L23 A13 L22 A12 L21 | L25 A16 L26 A17 L27 A18 L28 A19
extrude "Выдавливание16" cut sketch "Эскиз12" against normal blind 4 contours A0 | A1 | A2 | A3
extrude "Выдавливание19" cut sketch "Эскиз13" along normal blind 45 contours L13 E11 L10 E13 L14 L65 | L66 L41 E33 L55 E35 L47
